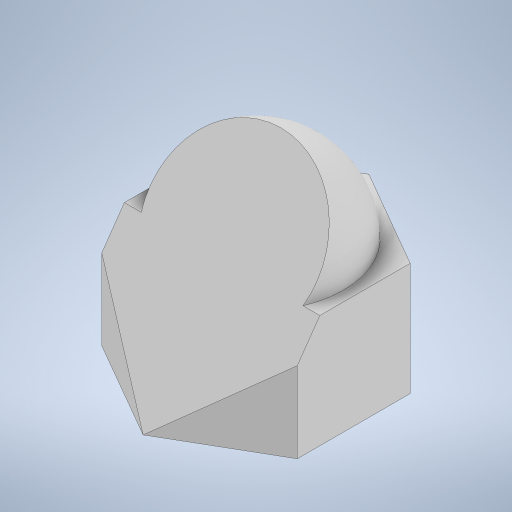
# Autodesk Inventor part: Деталь1
Saved by Autodesk Inventor 2024 (Build 280153000, 153)
## iProperties
Created: 2023-11-10
Part Number: Деталь1
Material: Типовые
Document SubType Name: Modeling
Designer: User
Density: 1 g/cm^3
Appearance: По умолчанию
Author: User
Autodesk Inventor part; units mm, degrees
ref_plane "YZ Plane" through (0, 0, 0) normal (1, 0, 0) x (0, 1, 0)
ref_plane "XZ Plane" through (0, 0, 0) normal (0, 1, 0) x (-1, 0, 0)
ref_plane "XY Plane" through (0, 0, 0) normal (0, 0, 1) x (1, 0, 0)
sketch "Эскиз1" plane through (0, 0, 0) normal (0, 1, 0) x (-1, 0, 0)
  line L0 (0, -45) -> (-38.9711, -22.5)
  line L1 (-38.9711, -22.5) -> (-38.9711, 22.5)
  line L2 (-38.9711, 22.5) -> (0, 45)
  line L3 (0, 45) -> (38.9711, 22.5)
  line L4 (38.9711, 22.5) -> (38.9711, -22.5)
  line L5 (38.9711, -22.5) -> (0, -45)
  point P0 (0, 0)
  point P1 (0, 0)
  dimension "d2" = 45
  constraints: 12 end point, 1 coincident, 13 other
  measures "d2" distance of L0.start point (0, 0)
extrude "Выдавливание1" add sketch "Эскиз1" along normal blind 45
sketch "Эскиз3" plane through (0, 0, 0) normal (1, 0, 0) x (0, 1, 0)
  line L0 (45, -22.5) -> (45, 22.5) projected
  line L1 (45, 0) -> (80, 0)
  line L2 (45, 22.5) -> (45, -22.5) projected
  line L3 (45, 0) -> (45, -35)
  arc A0 (45, -35) -> (45, 35) centre (45, 0) ccw
  point P0 (0, 0)
  dimension "d3" = 35
  dimension "d4" = 35
  constraints: 4 end point, 2 midpoint, 2 point on circle, 1 centre point, 1 coincident, 1 horizontal, 1 point on line
  measures "d3" distance of L3.start L1.end
  measures "d4" distance of L3.end L1.start
revolve "Вращение1" add sketch "Эскиз3" angle 360 about axis through (0, 45, 0) along (0, 1, 0)
sketch "Эскиз5" plane through (0, 0, 0) normal (1, 0, 0) x (0, 1, 0)
  arc A0 (45, -35) -> (45, 35) centre (45, 0) ccw projected
  line L0 (0, 22.5) -> (0, 45) projected
  line L1 (77.2198, 45) -> (0, 45)
  line L2 (97.7076, -23.3946) -> (97.7076, 45.0272)
  line L3 (97.7076, 45.0272) -> (76.0865, 45)
  line L4 (97.7076, -23.3946) -> (0, 45)
  point P0 (0, 0)
  point P1 (78.541, -10)
  point P2 (80, 0)
  dimension "d6" = 10
  constraints: 8 end point, 2 point on circle, 1 perpendicular, 1 point on line, 1 vertical
  measures "d6" vertical distance of point (80, 0) point (78.541, -10)
extrude "Выдавливание2" cut sketch "Эскиз5" along normal blind 100 and the other way blind 100
